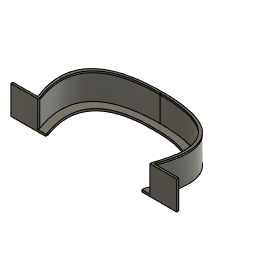
WS v1 v5 release (Autodesk Fusion 360 design; units mm, degrees)
Autodesk Fusion 360 part; units mm, degrees
sketch "Sketch16" plane through (0, 0, 0) normal (0, 1, 0) x (1, 0, 0)
  spline S0 degree 2 poles (35, 108.9313) (51, 148.9313) (0, 148.9313) knots 0 0 0 6.568937 6.568937 6.568937
  spline S1 degree 2 poles (-35, 108.9313) (-51, 148.9313) (0, 148.9313) knots 0 0 0 6.568937 6.568937 6.568937
  spline S2 degree 2 poles (-35, 108.9313) (-51, 148.9313) (0, 148.9313) knots 0 0 0 6.568937 6.568937 6.568937
  spline S3 degree 2 poles (35, 108.9313) (51, 148.9313) (0, 148.9313) knots 0 0 0 6.568937 6.568937 6.568937
  line L0 (-35, 108.9313) -> (-50, 108.9313)
  line L1 (35, 108.9313) -> (50, 108.9313)
  spline S4 degree 2 poles (-33.7996, 108.9313) (-48.6, 147.7313) (0, 147.7) knots 0 0 0 6.326066 6.326066 6.326066
  spline S5 degree 2 poles (33.7996, 108.9313) (48.6, 147.7313) (0, 147.7) knots 0 0 0 6.326066 6.326066 6.326066
  line L2 (-50, 108.9313) -> (-50, 107.7313)
  line L3 (33.7996, 108.9313) -> (33.7996, 107.7313)
  line L4 (50, 108.9313) -> (50, 107.7313)
  line L5 (33.7996, 107.7313) -> (50, 107.7313)
  line L6 (-33.7996, 108.9313) -> (-33.7996, 107.7313)
  line L7 (-50, 107.7313) -> (-33.7996, 107.7313)
  spline S6 degree 2 poles (-28.9996, 108.9313) (-41.9895, 143.9861) (0, 143.5) knots 0 0 0 5.564752 5.564752 5.564752
  spline S7 degree 2 poles (28.9996, 108.9313) (41.9895, 143.9861) (0, 143.5) knots 0 0 0 5.564752 5.564752 5.564752
  line L8 (-33.7996, 107.7313) -> (-29, 107.7313)
  line L9 (-29, 107.7313) -> (-28.9996, 108.9313)
  line L10 (28.9996, 108.9313) -> (28.9996, 107.7313)
  line L11 (28.9996, 107.7313) -> (33.7996, 107.7313)
  spline S8 degree 2 poles (-33.7996, 108.9313) (-48.6, 147.7313) (0, 147.7) knots 0 0 0 6.326066 6.326066 6.326066
  line L12 (-33.7996, 108.9313) -> (-33.7996, 107.7313)
  line L13 (-33.7996, 107.7313) -> (-29, 107.7313)
  spline S9 degree 2 poles (33.7996, 108.9313) (48.6, 147.7313) (0, 147.7) knots 0 0 0 6.326066 6.326066 6.326066
  line L14 (33.7996, 108.9313) -> (33.7996, 107.7313)
  line L15 (28.9996, 107.7313) -> (33.7996, 107.7313)
  spline S10 degree 2 poles (-33.7996, 108.9313) (-48.6, 147.7313) (0, 147.7) knots 0 0 0 6.326066 6.326066 6.326066
  line L16 (-33.7996, 108.9313) -> (-33.7996, 107.7313)
  line L17 (-33.7996, 107.7313) -> (-29, 107.7313)
  spline S11 degree 2 poles (33.7996, 108.9313) (48.6, 147.7313) (0, 147.7) knots 0 0 0 6.326066 6.326066 6.326066
  line L18 (33.7996, 108.9313) -> (33.7996, 107.7313)
  line L19 (28.9996, 107.7313) -> (33.7996, 107.7313)
  spline S12 degree 2 poles (-33.7996, 158.9313) (-56.6, 197.7313) (0, 197.7) knots 0 0 0 6.72439 6.72439 6.72439
  line L20 (-33.7996, 158.9313) -> (-33.7996, 157.7313)
  line L21 (-33.7996, 157.7313) -> (-29, 157.7313)
  spline S13 degree 2 poles (33.7996, 158.9313) (56.6, 197.7313) (0, 197.7) knots 0 0 0 6.72439 6.72439 6.72439
  line L22 (33.7996, 158.9313) -> (33.7996, 157.7313)
  line L23 (28.9996, 157.7313) -> (33.7996, 157.7313)
  line L24 (-29, 157.7313) -> (28.9996, 157.7313)
  line L25 (-0.0002, 107.7313) -> (-0.0002, 127.7313)
  dimension "d103" = 15
  dimension "d104" = 15
  dimension "d105" = 1.2
  dimension "d106" = 1.2
  dimension "d107" = 1.2
  dimension "d108" = 1.2
  dimension "d115" = 1.2
  dimension "d116" = 1.2
  dimension "d117" = 1.2
  dimension "d118" = 1.2
  dimension "d119" = 1.2
  dimension "d120" = 1.2
  dimension "d123" = 20
  constraint perpendicular L0 L2
  constraint vertical L3
  constraint perpendicular L1 L4
  constraint perpendicular L4 L5
  constraint perpendicular L0 L6
  constraint perpendicular L6 L7
  constraint perpendicular L6 L8
  constraint perpendicular L5 L10
  constraint perpendicular L3 L11
  constraint vertical L14
  constraint perpendicular L12 L13
  constraint perpendicular L14 L15
  constraint vertical L18
  constraint perpendicular L16 L17
  constraint perpendicular L18 L19
  constraint vertical L22
  constraint perpendicular L20 L21
  constraint perpendicular L22 L23
  constraint parallel L23 L24
  measures "d103" distance of S1.start L0.end
  measures "d104" distance of S0.start L1.end
  measures "d105" distance of L0.end L2.end
  measures "d106" distance of S5.start L3.end
  measures "d107" distance of L1.end L4.end
  measures "d108" distance of S4.start L6.end
  measures "d115" distance of S5.start L3.end
  measures "d116" distance of L6.end S4.start
  measures "d117" distance of S5.start L3.end
  measures "d118" distance of L6.end S4.start
  measures "d119" distance of S13.start L22.end
  measures "d120" distance of L20.end S12.start
  measures "d123" distance of L25.start L25.end
extrude "Extrude17" add sketch "Sketch16" along normal blind 17.4 contours S0 S1 S2 S3 L0 L1 S4 S5 L2 L3 L4 L5 L6 L7 S8 L12 S9 L14 S10 L16 S11 L18 makes body 1
extrude "Extrude18" add sketch "Sketch16" along normal blind 1.2 contours S4 S5 L3 L6 S6 S7 L8 L9 L10 L11 S8 L12 L13 S9 L14 L15 S10 L16 L17 S11 L18 L19 bodies 1
extrude "Extrude19" cut 1 faces at (-38.2206, 17.4, -125.4141) along direction (0, -1, 0) blind 1.2 on bodies 1 bodies 1
extrude "Extrude20" add sketch "Sketch16" along normal blind 15 separate body contours S12 L20 L21 S13 L22 L23 L24 makes body 2
move_body "Move2" [no effect]
move_body "Move3" bodies 1 to x (1, 0, 0) y (0, 1, 0) z (0, 0, 1) at (-1.1592, 0, 104.3758)
extrude "Extrude21" add 1 faces at (-39.3798, 16.2, -21.0383) along direction (0, 1, 0) blind 1 on bodies 1 bodies 1
hidden bodies 2
